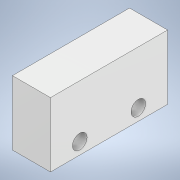
# Autodesk Inventor part: Stop_sw
Saved by Autodesk Inventor 2020 (Build 240168000, 168)
## iProperties
Created: 2022-03-21
Part Number: Stop_sw
Material: Tworzywo sztuczne ABS
Document SubType Name: Modeling
Designer: mikoma
Density: 1.06 g/cm^3
Appearance: Gładki — biały
Mass: 1.44816 g
Surface Area: 9.25467 cm^2
Volume: 1.36619 cm^3
Author: mikoma
Autodesk Inventor part; units mm, degrees
ref_plane "YZ Plane" through (0, 0, 0) normal (1, 0, 0) x (0, 1, 0)
ref_plane "XZ Plane" through (0, 0, 0) normal (0, 1, 0) x (-1, 0, 0)
ref_plane "XY Plane" through (0, 0, 0) normal (0, 0, 1) x (1, 0, 0)
sketch "Szkic1" plane through (0, 0, 0) normal (1, 0, 0) x (0, 1, 0)
  line L0 (-5.5, 10) -> (5.5, 10)
  line L1 (5.5, 10) -> (5.5, -10)
  line L2 (5.5, -10) -> (-5.5, -10)
  line L3 (-5.5, -10) -> (-5.5, 10)
  line L4 (-5.5, 10) -> (5.5, -10) construction
  line L5 (5.5, 10) -> (-5.5, -10) construction
  point P0 (0, 0)
  dimension "d0" = 20
  dimension "d1" = 11
  constraints: 12 end point, 2 midpoint, 2 parallel, 1 horizontal, 1 perpendicular
  measures "d0" distance of L0.end L1.end
  measures "d1" distance of L1.end L2.end
extrude "Wyciągnięcie proste1" add sketch "Szkic1" along normal blind 6.5
sketch "Szkic2" plane through (6.5, 0, 0) normal (1, 0, 0) x (0, 0, -1)
  line L0 (-9.9535, -3.5) -> (10, -3.5) construction
  line L1 (10, -5.5) -> (10, 5.5) projected
  line L2 (-10, -5.5) -> (10, -5.5) projected
  circle A0 centre (-5, -3.5) radius 1.25
  circle A1 centre (5, -3.5) radius 1.25
  line L3 (-10, 5.5) -> (-10, -5.5) projected
  point P0 (0, 0)
  dimension "d4" = 2
  dimension "d5" = 5
  dimension "d6" = 5
  dimension "d7" = 2.5
  dimension "d8" = 2.5
  constraints: 3 point on line, 2 centre point, 2 end point, 1 horizontal
  measures "d4" distance between parallel lines of L2 L0
  measures "d5" distance from line of L3 A0.centre
  measures "d6" distance from line of L1 A1.centre
  measures "d7" diameter of A0
  measures "d8" diameter of A1
extrude "Wyciągnięcie proste2" cut sketch "Szkic2" against normal through all
